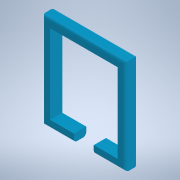
# Autodesk Inventor part: BumperSub
Saved by Autodesk Inventor 2020 (Build 240168000, 168)
## iProperties
Created: 2020-01-19
Part Number: BumperSub
Material: Generic
Document SubType Name: Modeling
Designer: srini
Density: 1 g/cm^3
Appearance: Sky Blue Dark
Author: srini
Autodesk Inventor part; units mm, degrees
ref_plane "YZ Plane" through (0, 0, 0) normal (1, 0, 0) x (0, 1, 0)
ref_plane "XZ Plane" through (0, 0, 0) normal (0, 1, 0) x (-1, 0, 0)
ref_plane "XY Plane" through (0, 0, 0) normal (0, 0, 1) x (1, 0, 0)
sketch "Sketch1" plane through (0, 0, 0) normal (0, 0, 1) x (1, 0, 0)
  line L0 (787.4, -34.925) -> (547.2722, -34.925) construction
  line L1 (793.75, -30.988) -> (793.75, 781.812) construction
  line L2 (787.4, 785.749) -> (101.6, 785.749) construction
  line L3 (95.25, 781.812) -> (95.25, -30.988) construction
  line L4 (795.3375, -36.5125) -> (93.6625, -36.5125)
  line L5 (93.6625, -36.5125) -> (93.6625, 787.3365)
  line L6 (93.6625, 787.3365) -> (795.3375, 787.3365)
  line L7 (795.3375, 787.3365) -> (795.3375, -36.5125)
  line L8 (877.8875, -119.0625) -> (11.1125, -119.0625)
  line L9 (11.1125, -119.0625) -> (11.1125, 869.8865)
  line L10 (11.1125, 869.8865) -> (877.8875, 869.8865)
  line L11 (877.8875, 869.8865) -> (877.8875, -119.0625)
  point P0 (0, 0)
  dimension "d0" = 1.5875
  dimension "d1" = 1.5875
  dimension "d2" = 1.5875
  dimension "d3" = 1.5875
  dimension "d4" = 82.55
  constraints: 16 end point, 4 parallel, 2 perpendicular, 1 horizontal, 3 other
  measures "d0" distance between parallel lines of L2 L6
  measures "d1" distance between parallel lines of L3 L5
  measures "d2" distance between parallel lines of L0 L4
  measures "d3" distance between parallel lines of L1 L7
  measures "d4" distance between parallel lines of L7 L11
extrude "Extrusion1" add sketch "Sketch1" against normal blind 127
fillet "Fillet1" radius 31.75 8 edges at (444.5, -119.0625, -127) (444.5, -119.0625, 0) (11.1125, 375.412, 0) (11.1125, 375.412, -127) (444.5, 869.8865, -127) (444.5, 869.8865, 0) (877.8875, 375.412, -127) (877.8875, 375.412, 0)
sketch "Sketch2" plane through (0, 0, -127) normal (0, 0, -1) x (-1, 0, 0)
  line L0 (-547.2722, -247.9153) -> (-341.7278, -247.9153)
  line L1 (-341.7278, -247.9153) -> (-341.7278, 127.868)
  line L2 (-341.7278, 127.868) -> (-547.2722, 127.868)
  line L3 (-547.2722, 127.868) -> (-547.2722, -247.9153)
  line L4 (-547.2722, -34.925) -> (-548.4674, -30.988) projected
  line L5 (-341.7278, -34.925) -> (-340.5326, -30.988) projected
  point P0 (0, 0)
  constraints: 8 end point, 2 parallel, 2 point on line, 1 horizontal, 1 perpendicular
extrude "Extrusion2" cut sketch "Sketch2" against normal through all
equation "\"d1\" = d0"
equation "\"d2\" = d0"
equation "\"d3\" = d0"
body "Solid1"
